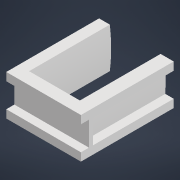
# Autodesk Inventor part: Coils
Saved by Autodesk Inventor 2022.4 (Build 264492010, 492A)
## iProperties
Created: 2023-10-10
Part Number: Coils
Material: Stainless Steel
Document SubType Name: Modeling
Designer: Harsh
Density: 8 g/cm^3
Appearance: Semi-Polished
Author: Harsh
Autodesk Inventor part; units mm, degrees
ref_plane "YZ Plane" through (0, 0, 0) normal (1, 0, 0) x (0, 1, 0)
ref_plane "XZ Plane" through (0, 0, 0) normal (0, 1, 0) x (-1, 0, 0)
ref_plane "XY Plane" through (0, 0, 0) normal (0, 0, 1) x (1, 0, 0)
sketch "Sketch1" plane through (0, 0, 0) normal (0, 0, 1) x (1, 0, 0)
  line L0 (0, 0) -> (50, 0) construction
  line L1 (0, 0) -> (37.5, 0)
  line L2 (37.5, 0) -> (34.5, 0)
  line L3 (34.5, 0) -> (34.5, 5)
  line L4 (34.5, 5) -> (53, 5)
  line L5 (53, 5) -> (53, -5)
  line L6 (53, -5) -> (34.5, -5)
  line L7 (34.5, -5) -> (34.5, 5)
  line L8 (0, 0) -> (37.1652, 5) construction
  line L9 (0, 0) -> (37.1652, -5) construction
  arc A0 (37.1652, -5) -> (37.1652, 5) centre (0, 0) ccw
  line L10 (0, 0) -> (49.7494, 5) construction
  arc A1 (49.7494, -5) -> (49.7494, 5) centre (0, 0) ccw
  line L11 (34.5, -5) -> (53, -5)
  line L12 (53, -5) -> (53, -3)
  line L13 (53, -3) -> (34.5, -3)
  line L14 (34.5, -3) -> (34.5, -5)
  line L15 (34.5, 5) -> (53, 5)
  line L16 (53, 5) -> (53, 3)
  line L17 (53, 3) -> (34.5, 3)
  line L18 (34.5, 3) -> (34.5, 5)
  line L19 (37.1652, -5) -> (36.1652, -5)
  arc A2 (36.1652, -5) -> (36.1652, 5) centre (-1, 0) ccw
  line L20 (49.7494, -5) -> (50.7494, -5)
  arc A3 (50.7494, -5) -> (50.7494, 5) centre (1, 0) ccw
  point P0 (36.3798, 3)
  point P1 (36.3798, -3)
  point P2 (50.9099, -3)
  point P3 (50.9099, 3)
  dimension "d7" = 50
  dimension "d8" = 37.5
  dimension "d9" = 3
  dimension "d10" = 5
  dimension "d11" = 18.5
  dimension "d12" = 10
  dimension "d13" = 37.5
  dimension "d14" = 50
  dimension "d15" = 2
  dimension "d16" = 2
  dimension "d17" = 1
  dimension "d18" = 1
  constraints: 42 end point, 10 point on circle, 9 point on line, 6 parallel, 4 centre point, 4 horizontal, 4 perpendicular, 1 symmetric about line
  measures "d7" distance of L0.start L0.end
  measures "d8" distance of L0.start L1.end
  measures "d9" distance of L1.end L2.end
  measures "d10" distance of L2.end L3.end
  measures "d11" distance of L5.end L6.end
  measures "d12" distance of L4.end L5.end
  measures "d13" distance of L0.start L8.end
  measures "d14" distance of L10.start L10.end
  measures "d15" distance of L12.end L11.end
  measures "d16" distance of L15.end L16.end
  measures "d17" distance of L9.end L19.end
  measures "d18" distance of L20.start L20.end
extrude "Extrusion1" add sketch "Sketch1" along normal blind 1
extrude "Extrusion2" add sketch "Sketch1" along normal blind 3 contours L3 L4 A2 L17 | L13 A2 L6 L7 | L13 A0 L6 A2 | A2 L4 A0 L17 | L13 A1 L6 A0 | A0 L4 A1 L17 | L13 A3 L6 A1 | A1 L4 A3 L17 | L13 L5 L6 A3 | A3 L4 L5 L17
extrude "Extrusion3" add sketch "Sketch1" against normal blind 20 contours A2 L17 A0 L1 | L1 A0 L13 A2 | L3 L4 A2 L17 | L13 A2 L6 L7 | L13 A0 L6 A2 | A2 L4 A0 L17 | L13 A3 L6 A1 | A1 L17 A3 L13 | A1 L4 A3 L17 | L13 L5 L6 A3 | A3 L4 L5 L17
body "Solid1"
